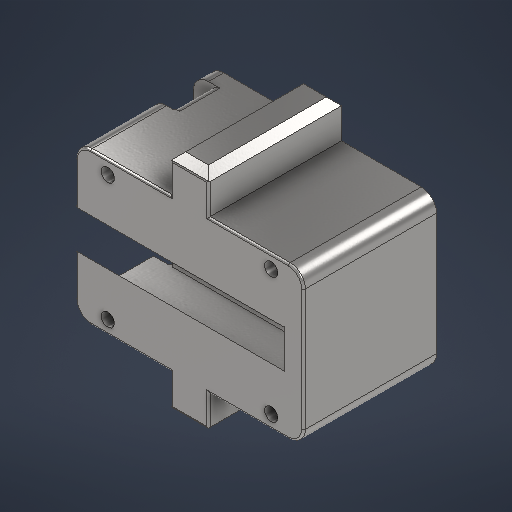
# Autodesk Inventor part: Wrist
Saved by Autodesk Inventor 2025.2 (Build 292293000, 293)
## iProperties
Created: 2025-06-16
Part Number: Wrist
Material: PLA Plastic
Document SubType Name: Modeling
Designer: Tiago
Density: 1.18 g/cm^3
Appearance: Galvanized
Mass: 52.1514 g
Surface Area: 188.625 cm^2
Volume: 44.1961 cm^3
Author: Tiago
Autodesk Inventor part; units mm, degrees
ref_plane "YZ Plane" through (0, 0, 0) normal (1, 0, 0) x (0, 1, 0)
ref_plane "XZ Plane" through (0, 0, 0) normal (0, 1, 0) x (-1, 0, 0)
ref_plane "XY Plane" through (0, 0, 0) normal (0, 0, 1) x (1, 0, 0)
sketch "Sketch1" plane through (0, 0, 0) normal (0, 0, 1) x (1, 0, 0)
  line L0 (-26, -20) -> (26, -20)
  line L1 (30, -16) -> (30, 16)
  line L2 (26, 20) -> (-26, 20)
  line L3 (-30, 16) -> (-30, -16)
  arc A0 (30, 16) -> (26, 20) centre (26, 16) ccw
  arc A1 (-26, 20) -> (-30, 16) centre (-26, 16) ccw
  arc A2 (-30, -16) -> (-26, -20) centre (-26, -16) ccw
  arc A3 (26, -20) -> (30, -16) centre (26, -16) ccw
  line L4 (-25, 13) -> (30, 13)
  line L5 (-25, -13) -> (30, -13)
  line L6 (22, -13) -> (22, 13)
  line L7 (-22, -13) -> (-22, 13)
  circle A4 centre (0, 0) radius 4.05
  circle A5 centre (16, 0) radius 1.75
  circle A6 centre (-16, 0) radius 1.75
  line L8 (25, 20) -> (25, -20)
  point P0 (-30, -20)
  point P1 (30, 20)
  point P2 (30, -20)
  point P3 (-30, 20)
  point P4 (30, 0)
  point P5 (0, 20)
  dimension "d0" = 60
  dimension "d1" = 40
  dimension "d4" = 4
  dimension "d7" = 13
  dimension "d8" = 13
  dimension "d9" = 22
  dimension "d10" = 22
  dimension "d14" = 8.1
  dimension "d15" = 3.5
  dimension "fu" = 3.5
  dimension "d17" = 16
  dimension "d18" = 16
  dimension "d94" = 5
  constraints: 18 end point, 14 point on line, 8 point on circle, 8 tangent, 7 centre point, 4 perpendicular, 3 coincident, 3 equal radius, 3 horizontal alignment, 2 horizontal, 2 midpoint, 2 parallel, 1 vertical, 1 vertical alignment
  measures "d0" distance of point (-30, -20) point (30, -20)
  measures "d1" distance of point (30, -20) point (30, 20)
  measures "d4" radius of A0
  measures "d7" distance from line of L4 point (0, 0)
  measures "d8" distance from line of point (0, 0) L5
  measures "d9" distance from line of point (0, 0) L6
  measures "d10" distance from line of point (0, 0) L7
  measures "d14" diameter of A4
  measures "d15" diameter of A5
  measures "fu" diameter of A6
  measures "d17" distance of point (0, 0) A5.centre
  measures "d18" distance of point (0, 0) A6.centre
  measures "d94" distance between parallel lines of L1 L8
extrude "Extrusion1" add sketch "Sketch1" along normal blind 4
ref_plane "Work Plane3" through (0, 0, 15) normal (0, 0, 1) x (1, 0, 0)
sketch "Sketch2" plane through (0, 0, 15) normal (0, 0, 1) x (1, 0, 0)
  line L0 (-25, -13) -> (25, -13)
  line L1 (-25, -13) -> (-25, -20)
  line L2 (-25, -20) -> (25, -20)
  line L3 (25, -20) -> (25, -13)
  line L4 (-2.1814, 0) -> (2.1814, 0) construction
  line L5 (-25, 13) -> (25, 13)
  line L6 (-25, 13) -> (-25, 20)
  line L7 (-25, 20) -> (25, 20)
  line L8 (25, 20) -> (25, 13)
  point P0 (0, 0)
  point P1 (0, -13)
  point P2 (25, -20)
  point P3 (25, -20)
  point P4 (0, 0)
  point P5 (0, 13)
  point P6 (25, 20)
  point P7 (25, 20)
  dimension "d38" = 0
  dimension "d34" = 50
  dimension "d35" = 13
  dimension "d36" = 7
  dimension "d37" = 50
  constraints: 18 end point, 11 symmetric about line, 8 point on line, 6 horizontal, 3 vertical, 2 coincident, 2 midpoint, 1 perpendicular, 1 vertical alignment, 16 other
  measures "d34" distance of L0.start L0.end
  measures "d35" distance from line of point (0, 0) L0
  measures "d36" distance of L0.start point (-25, -20)
  measures "d37" distance of point (-25, -20) point (25, -20)
ref_plane "Work Plane1" through (0, 0, 25) normal (0, 0, 1) x (1, 0, 0)
sketch "Sketch3" plane through (0, 0, 25) normal (0, 0, 1) x (1, 0, 0)
  line L0 (-30, -5) -> (30, -5)
  line L1 (30, -5) -> (30, -16)
  line L2 (26, -20) -> (-26, -20)
  line L3 (-30, -16) -> (-30, -5)
  line L4 (-3.5121, 0) -> (3.5121, 0) construction
  arc A0 (26, -20) -> (30, -16) centre (26, -16) ccw
  arc A1 (-30, -16) -> (-26, -20) centre (-26, -16) ccw
  line L5 (-30, 5) -> (30, 5)
  line L6 (30, 5) -> (30, 16)
  line L7 (26, 20) -> (-26, 20)
  line L8 (-30, 16) -> (-30, 5)
  arc A2 (30, 16) -> (26, 20) centre (26, 16) ccw
  arc A3 (-26, 20) -> (-30, 16) centre (-26, 16) ccw
  point P0 (0, 0)
  point P1 (0, -5)
  point P2 (30, -20)
  point P3 (-30, -20)
  point P4 (0, 0)
  point P5 (0, 5)
  point P6 (30, 20)
  point P7 (-30, 20)
  dimension "d25" = 5
  dimension "d26" = 15
  dimension "d27" = 60
  dimension "d28" = 4
  dimension "d29" = 5
  dimension "d62" = 15
  dimension "d63" = 60
  constraints: 18 end point, 11 symmetric about line, 8 point on circle, 8 point on line, 4 centre point, 4 tangent, 2 coincident, 2 horizontal, 2 midpoint, 1 equal radius, 1 perpendicular, 1 vertical, 1 vertical alignment, 2 other
  measures "d25" distance from line of point (0, 0) L0
  measures "d26" distance of L0.end point (30, -20)
  measures "d27" distance of point (30, -20) point (-30, -20)
  measures "d28" radius of A0
  measures "d29" distance from line of L5 point (0, 0)
  measures "d62" distance from line of L2 L0.start
  measures "d63" distance between parallel lines of L6 L8
ref_plane "Work Plane2" through (0, 0, 15) normal (0, 0, 1) x (1, 0, 0)
extrude "Extrusion3" add sketch "Sketch3" along normal blind 10 and the other way blind 10
extrude "Extrusion5" add sketch "Sketch2" against normal up to surface (11 mm away)
sketch "Sketch8" plane through (-30, 5, 35) normal (-1, 0, 0) x (0, 0, 1)
  line L0 (-20, -10) -> (0, -10) projected
  line L1 (0, -10) -> (0, -21) projected
  line L2 (0, 11) -> (0, 0) projected
  line L3 (0, 0) -> (-20, 0) projected
  line L4 (-20, 11) -> (0, 11) projected
  line L5 (-31, 11) -> (-31, -21) projected
  line L6 (-35, 11) -> (-31, 11) projected
  line L7 (-19.5, 0) -> (0, 0)
  line L8 (-20, 15) -> (-20, 8) projected
  line L9 (0, 0) -> (-15.9217, 15.9217)
  line L10 (0, -10) -> (-19.5, -29.5)
  line L11 (-19.5, -29.5) -> (-19.5, -10)
  line L12 (-10, -19.75) -> (-20, -19.75) projected
  line L13 (-19.5, -10) -> (0, -10)
  line L14 (-19.5, 0) -> (-20, 0)
  line L15 (-20, 0) -> (-20, 11.547)
  line L16 (-20, 11.547) -> (-15.9217, 15.9217)
  line L17 (-19.5, -29.5) -> (-20, -21.547)
  line L18 (-20, -21.547) -> (-20, -10)
  line L19 (-20, -10) -> (-19.5, -10)
  line L20 (-20, -21) -> (0, -21) projected
  line L21 (-20, -21) -> (-20, -10) projected
  line L22 (-20, 0) -> (-20, 11) projected
  line L23 (-35, -21) -> (-31, -21) projected
  line L24 (-35, -21) -> (-35, 11) projected
  point P0 (-35, -5)
  point P1 (-16.8875, -19.75)
  point P2 (-11, 11)
  point P3 (-11, -21)
  point P4 (-19.5, -21)
  point P5 (-19.5, -19.75)
  dimension "d71" = 45
  dimension "d72" = 45
  constraints: 22 end point, 5 perpendicular, 3 point on line
  measures "d71" angle of L3 L9
  measures "d72" angle of L0 L10
extrude "Extrusion6" cut sketch "Sketch8" against normal up to surface (60 mm away) contours L0 L11 L12 L18 | L0 L10 L20 L11 | L12 L11 L20 L18 | L3 L15 L8 L4 L9
chamfer "Chamfer3" distance 0.4 angle 45 2 edges at (0, 13, 15) (0, -13, 15)
sketch "Sketch9" plane through (-26, -20, 0) normal (0, -1, 0) x (1, 0, 0)
  line L0 (52, 0) -> (0, 0) projected
  line L1 (0, 35) -> (52, 35) projected
  line L2 (21, 0) -> (31, 0)
  line L3 (31, 0) -> (31, 35)
  line L4 (31, 35) -> (21, 35)
  line L5 (21, 35) -> (21, 0)
  point P0 (26, 0)
  point P1 (26, 35)
  dimension "d78" = 10
  dimension "d79" = 26
  constraints: 8 end point, 2 parallel, 2 point on line, 1 horizontal, 1 midpoint, 1 perpendicular
  measures "d78" distance between parallel lines of L5 L3
  measures "d79" horizontal distance of L0.end point (26, 35)
extrude "Extrusion7" add sketch "Sketch9" along normal blind 10
mirror "Mirror1" about plane through (0, 0, 0) normal (0, 1, 0) of "Extrusion7"
chamfer "Chamfer4" distance 2 angle 45 8 edges at (-5, -30, 17.5) (5, -30, 17.5) (-5, 30, 17.5) (5, 30, 17.5) (0, 30, 35) (0, -30, 35) (0, 30, 0) (0, -30, 0)
sketch "Sketch10" plane through (0, 0, 35) normal (0, 0, 1) x (1, 0, 0)
  line L0 (-5, 28) -> (5, 28) projected
  line L1 (5, 28) -> (5, 20) projected
  line L2 (5, 20) -> (26, 20) projected
  arc A0 (30, 16) -> (26, 20) centre (26, 16) ccw projected
  line L3 (30, 16) -> (30, 5) projected
  line L4 (30, 5) -> (-30, 5) projected
  line L5 (-30, 5) -> (-30, 16) projected
  arc A1 (-26, 20) -> (-30, 16) centre (-26, 16) ccw projected
  line L6 (-26, 20) -> (-5, 20) projected
  line L7 (-5, 20) -> (-5, 28) projected
  line L8 (5, -28) -> (-5, -28) projected
  line L9 (-5, -28) -> (-5, -20) projected
  line L10 (-5, -20) -> (-26, -20) projected
  arc A2 (-30, -16) -> (-26, -20) centre (-26, -16) ccw projected
  line L11 (-30, -16) -> (-30, -5) projected
  line L12 (-30, -5) -> (30, -5) projected
  line L13 (30, -5) -> (30, -16) projected
  arc A3 (26, -20) -> (30, -16) centre (26, -16) ccw projected
  line L14 (26, -20) -> (5, -20) projected
  line L15 (5, -20) -> (5, -28) projected
  arc A4 (-23.2494, 16.547) -> (-19.7506, 16.547) centre (-21.5, 16.5) ccw projected
  circle A5 centre (-21.5, 16.5) radius 1.75
  arc A6 (-23.2494, -16.547) -> (-19.7506, -16.547) centre (-21.5, -16.5) ccw projected
  circle A7 centre (-21.5, -16.5) radius 1.75
  circle A8 centre (21.5, -16.5) radius 1.75 projected
  circle A9 centre (21.5, -16.5) radius 1.75
  circle A10 centre (21.5, 16.5) radius 1.75 projected
  circle A11 centre (21.5, 16.5) radius 1.75
  point P0 (0, 0)
  dimension "d85" = 3.5
  dimension "d86" = 43
  dimension "d89" = 8.5
  dimension "d90" = 3.5
  dimension "d91" = 3.5
  dimension "d92" = 8.5
  constraints: 4 coincident, 3 centre point, 1 horizontal alignment, 1 vertical alignment, 3 other
  measures "d85" diameter of A5
  measures "d86" distance of point (-21.5, -16.5) A9.centre
  measures "d89" distance from line of L5 A5.centre
  measures "d90" distance from line of L6 A5.centre
  measures "d91" distance from line of L2 A11.centre
  measures "d92" distance from line of L3 A11.centre
extrude "Extrusion8" cut sketch "Sketch10" against normal blind 9 contours A5 A4 | A7 A6 | A8 | A10
ref_plane "Work Plane4" through (0, 0, 17.5) normal (0, 0, 1) x (1, 0, 0)
mirror "Mirror2" about plane through (0, 0, 17.5) normal (0, 0, 1) of "Extrusion8"
fillet "Fillet5" radius 0.5 18 edges at (-28.8284, 18.8284, 35) (-30, 10.5, 35) (-15.5, 20, 35) (28.8284, 18.8284, 35) (30, 10.5, 35) (15.5, 20, 35) (-5, 24, 35) (0, 28, 35) (5, 24, 35) (-28.8284, -18.8284, 35) (-15.5, -20, 35) (-30, -10.5, 35) (-5, -24, 35) (0, -28, 35) (5, -24, 35) (28.8284, -18.8284, 35) (30, -10.5, 35) (15.5, -20, 35)
extrude "Extrusion9" add sketch "Sketch1" along normal blind 35 contours L8 L5 L1 A3 L0 | L8 L4 L1 L5 | L8 L2 A0 L1 L4
fillet "Fillet6" radius 0.5 5 edges at (28.8284, 18.8284, 35) (25.5, 20, 35) (28.8284, -18.8284, 35) (25.5, -20, 35) (30, 0, 35)
fillet "Fillet7" radius 2 2 edges at (-25, 20, 9.5) (-25, -20, 9.5)
chamfer "Chamfer5" distance 0.5 angle 45 8 edges at (-30, 16, 19.5) (-30, -16, 19.5) (-25, 14.7, 15) (-25, -14.7, 15) (-25, -17, 15) (-24.4142, -19.4142, 15) (-25, 17, 15) (-24.4142, 19.4142, 15)
equation "\"d15\" = fu"
body "Solid1"
